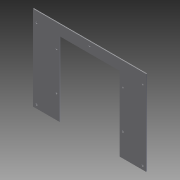
# Autodesk Inventor part: top plate
Saved by Autodesk Inventor 2011 SP1 (Build 150282100, 282)
## iProperties
Created: 2012-01-20
Part Number: top plate
Document SubType Name: Modeling
Designer: Christopher
Density: 1 g/cm^3
Author: Christopher
Autodesk Inventor part; units mm, degrees
ref_plane "YZ Plane" through (0, 0, 0) normal (1, 0, 0) x (0, 1, 0)
ref_plane "XZ Plane" through (0, 0, 0) normal (0, 1, 0) x (-1, 0, 0)
ref_plane "XY Plane" through (0, 0, 0) normal (0, 0, 1) x (1, 0, 0)
sketch "Sketch1" plane through (0, 0, 0) normal (0, 0, 1) x (1, 0, 0)
  line L0 (717.55, 0) -> (717.55, 304.8)
  line L1 (717.55, 304.8) -> (0, 304.8)
  line L2 (0, 304.8) -> (0, 0)
  line L3 (250.825, 0) -> (250.825, 266.7)
  line L4 (250.825, 266.7) -> (466.725, 266.7)
  line L5 (466.725, 266.7) -> (466.725, 0)
  line L6 (466.725, 0) -> (717.55, 0)
  line L7 (250.825, 0) -> (0, 0)
  point P0 (358.775, 152.4)
  point P1 (358.775, 289.941)
  point P2 (239.661, 221.1705)
  point P3 (239.661, 83.6295)
  point P4 (358.775, 14.859)
  point P5 (477.889, 83.6295)
  point P6 (477.889, 221.1705)
  point P7 (12.7, 266.7)
  point P8 (12.7, 12.7)
  point P9 (704.85, 12.7)
  point P10 (704.85, 266.7)
  dimension "d0" = 717.55
  dimension "d1" = 304.8
  dimension "d2" = 358.775
  dimension "d3" = 152.4
  dimension "d4" = 137.541
  dimension "d7" = 360
  dimension "d11" = 38.1
  dimension "d21" = 38.1
  dimension "d22" = 12.7
  dimension "d23" = 12.7
  dimension "d24" = 12.7
  dimension "d25" = 12.7
  dimension "d26" = 12.7
  dimension "d27" = 12.7
  dimension "d28" = 38.1
  dimension "d36" = 107.95
  dimension "d37" = 107.95
  constraints: 16 end point, 2 parallel, 2 perpendicular, 1 collinear, 7 other
  measures "d0" distance of L1.end L0.end
  measures "d1" distance of L0.end L0.start
  measures "d2" distance from line of L2 point (358.775, 152.4)
  measures "d3" distance from line of L1 point (358.775, 152.4)
  measures "d4" distance of point (358.775, 289.941) point (358.775, 152.4)
  measures "d11" distance between parallel lines of L1 L4
  measures "d21" distance from line of L1 point (12.7, 266.7)
  measures "d22" distance from line of L7 point (12.7, 12.7)
  measures "d23" distance from line of L2 point (12.7, 12.7)
  measures "d24" distance from line of L2 point (12.7, 266.7)
  measures "d25" distance from line of L0 point (704.85, 266.7)
  measures "d26" distance from line of L0 point (704.85, 12.7)
  measures "d27" distance from line of L6 point (704.85, 12.7)
  measures "d28" distance from line of L1 point (704.85, 266.7)
  measures "d36" distance from line of L3 point (358.775, 152.4)
  measures "d37" distance from line of point (358.775, 152.4) L5
extrude "Extrusion1" add sketch "Sketch1" against normal blind 3.175
hole "Hole1" at (358.775, 152.4, 0) at (358.775, 289.941, 0) at (239.661, 221.1705, 0) at (239.661, 83.6295, 0) at (358.775, 14.859, 0) at (477.889, 83.6295, 0) at (477.889, 221.1705, 0) direction (0, 0, -1) diameter 6.35 depth 25.4 tip angle 118
hole "Hole2" at (12.7, 266.7, 0) at (12.7, 12.7, 0) at (704.85, 12.7, 0) at (704.85, 266.7, 0) direction (0, 0, -1) diameter 6.35 depth 25.4 tip angle 118
body "Solid1"
